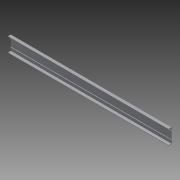
# Autodesk Inventor part: KR55-980-Protected Cover
Saved by Autodesk Inventor 2011 SP1 (Build 150282100, 282)
## iProperties
Created: 2013-10-23
Part Number: KR55-980-Protected Cover
Catalog Web Link: www.cadenas.de
Description: LM Guide Actuator - Protected Cover-KR
Vendor: THK
Document SubType Name: Modeling
Designer: PARTuser1
Manufacturer: THK
Density: 1 g/cm^3
Category: PARTsolutions
Company: THK
Title: KR55-980-Protected Cover
Author: Cadenas PARTsolutions
Comments: KR
PSOL_IDENT_0: {$CADENAS_DATA\23d-libs\thk\lm_guide_actuator\type_kr\parts\lm_g_a_kr_pc.prj},221 {VTYP=3D},{NB=KR55
PSOL_IDENT_1: -980-Protected Cover},{LINA=KR55-980-Protected Cover},{NN=LM Guide Actuator - Protected Cover},{DATE
PSOL_IDENT_2: =17.05.2010 06:32:41},{GEOMDATE=14.02.2008 10:19:00},{VERSION=},{LINEID=80},{LINESUBID=-1},{WBVAR=LM
PSOL_IDENT_3: }  {NB=KR55-980-Protected Cover},{LINA=KR55-980-Protected Cover},{KT=DUMMY},{ORDER=KR55},{TYPE=8.000
PSOL_IDENT_4: },{LM=980}
CNS_NT: KR
CNS_NB: KR55-980-Protected Cover
CNS_NBSYN: $ORDER.-$LM.-Protected Cover
CNS_LINA: KR55-980-Protected Cover
CNS_ORDER: KR55
CNS_TYPE: 8.000
CNS_LM: 980
SUPPLIER: THK
ARTICLENO: KR55-980-Protected Cover
BOMINFO: KR55-980-Protected Cover
CREATOR: CADENAS GmbH
Autodesk Inventor part; units mm, degrees
sketch "Sketch_1" plane through (0, 0, 0) normal (1, 0, 0) x (0, 1, 0)
  line L0 (16.5, 46) -> (1, 46)
  arc A0 (1, 46) -> (0, 45) centre (1, 45) ccw
  line L1 (0, 45) -> (0, 43)
  line L2 (0, 43) -> (17.5, 43)
  line L3 (17.5, 43) -> (17.5, 30)
  line L4 (17.5, 30) -> (14, 30)
  line L5 (14, 30) -> (14, 20)
  line L6 (14, 20) -> (17.5, 20)
  line L7 (17.5, 20) -> (17.5, -20)
  line L8 (17.5, -20) -> (14, -20)
  line L9 (14, -20) -> (14, -30)
  line L10 (14, -30) -> (17.5, -30)
  line L11 (17.5, -30) -> (17.5, -43)
  line L12 (17.5, -43) -> (0, -43)
  line L13 (0, -43) -> (0, -45)
  arc A1 (0, -45) -> (1, -46) centre (1, -45) ccw
  line L14 (1, -46) -> (16.5, -46)
  arc A2 (16.5, -46) -> (19.5, -43) centre (16.5, -43) ccw
  line L15 (19.5, -43) -> (19.5, 43)
  arc A3 (19.5, 43) -> (16.5, 46) centre (16.5, 43) ccw
  constraints: 32 end point, 8 point on circle, 4 centre point
extrude "Extrusion1" add sketch "Sketch_1" along normal blind 1010
sketch "Sketch_3" plane through (7.5, 0, 0) normal (1, 0, 0) x (0, 0, -1)
  line L0 (-25, 21.1) -> (-25, 19.5)
  line L1 (-25, 19.5) -> (-30, 19.5)
  line L2 (-30, 19.5) -> (-30, 20.1)
  line L3 (-30, 20.1) -> (-27.4, 20.5)
  line L4 (-27.4, 20.5) -> (-27.4, 21.1)
  line L5 (-27.4, 21.1) -> (-25, 21.1)
  line L6 (-25, 21.1) -> (-25, 19.5)
  constraints: 14 end point
revolve "Revolution1" add sketch "Sketch_3" angle 360 about axis through (7.5, 21.1, 25) along (0, 1, 0)
pattern_linear "Rectangular Pattern1" count 2 spacing 995 along (1, 0, 0) count 2 spacing 50 along (0, 0, -1) of "Revolution1"
ref_plane "pc_body_XY" through (7.5, 14, 0) normal (1, 0, 0) x (0, 0, -1)
ref_plane "pc_body_YZ" through (7.5, 14, 0) normal (0, 0, -1) x (0, 1, 0)
ref_plane "pc_body_ZX" through (7.5, 14, 0) normal (0, 1, 0) x (1, 0, 0)
body "Solid1"
